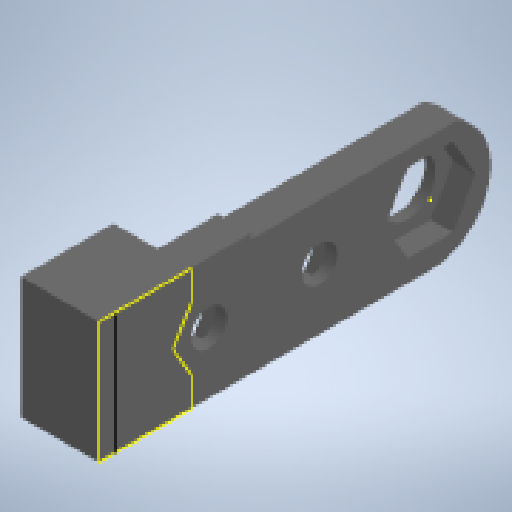
# Autodesk Inventor part: hand_finger_inside
Saved by Autodesk Inventor 2024.1 (Build 281209000, 209)
## iProperties
Created: 2025-01-23
Part Number: hand_finger_inside
Material: 一般
Document SubType Name: Modeling
Designer: hibik
Density: 1 g/cm^3
Appearance: 既定
Author: hibik
Autodesk Inventor part; units mm, degrees
ref_plane "YZ Plane" through (0, 0, 0) normal (1, 0, 0) x (0, 1, 0)
ref_plane "XZ Plane" through (0, 0, 0) normal (0, 1, 0) x (-1, 0, 0)
ref_plane "XY Plane" through (0, 0, 0) normal (0, 0, 1) x (1, 0, 0)
sketch "スケッチ1" plane through (0, 0, 0) normal (1, 0, 0) x (0, 1, 0)
  circle A0 centre (0, 0) radius 2.5
  line L0 (0, 4.0992) -> (3.55, 2.0496)
  line L1 (3.55, 2.0496) -> (3.55, -2.0496)
  line L2 (3.55, -2.0496) -> (0, -4.0992)
  line L3 (0, -4.0992) -> (-3.55, -2.0496)
  line L4 (-3.55, -2.0496) -> (-3.55, 2.0496)
  line L5 (-3.55, 2.0496) -> (0, 4.0992)
  circle A1 centre (0, 0) radius 5.5
  line L6 (5.5, 0) -> (-5.5, 0) construction
  line L7 (-5.5, 0) -> (-5.5, 30)
  line L8 (-5.5, 30) -> (5.5, 30)
  line L9 (5.5, 30) -> (5.5, 0)
  dimension "d2" = 11
  dimension "d0" = 5
  dimension "d1" = 7.1
  dimension "d3" = 30
  constraints: 20 end point, 3 coincident, 3 vertical, 2 parallel, 1 centre point, 1 horizontal, 1 perpendicular, 16 other
  measures "d0" diameter of A0
  measures "d1" distance between parallel lines of L4 L1
  measures "d3" distance of L8.end L6.start
extrude "押し出し1" add sketch "スケッチ1" along normal blind 3 contours A1 | A1 L7 L8 L9
extrude "押し出し2" add sketch "スケッチ1" along normal blind 1 contours L0 L1 L2 L3 L4 L5
sketch "スケッチ2" plane through (3, 0, 0) normal (1, 0, 0) x (0, 0, -1)
  circle A0 centre (-10, 0) radius 1.6
  circle A1 centre (-20, 0) radius 1.6
  point P0 (0, 0)
  dimension "d8" = 3.2
  dimension "d9" = 3.2
  dimension "d10" = 10
  dimension "d11" = 10
  constraints: 2 centre point, 2 horizontal alignment
  measures "d8" diameter of A0
  measures "d9" diameter of A1
  measures "d10" distance of point (0, 0) A0.centre
  measures "d11" distance of A1.centre A0.centre
extrude "押し出し3" cut sketch "スケッチ2" against normal through all
sketch "スケッチ3" plane through (0, 0, 0) normal (-1, 0, 0) x (0, 0, 1)
  circle A0 centre (20, 0) radius 1.6 projected
  circle A1 centre (10, 0) radius 1.6 projected
  line L0 (21.6454, -2.85) -> (18.3546, -2.85)
  line L1 (18.3546, -2.85) -> (16.7091, 0)
  line L2 (16.7091, 0) -> (18.3546, 2.85)
  line L3 (18.3546, 2.85) -> (21.6454, 2.85)
  line L4 (21.6454, 2.85) -> (23.2909, 0)
  line L5 (23.2909, 0) -> (21.6454, -2.85)
  line L6 (11.6454, -2.85) -> (8.3546, -2.85)
  line L7 (8.3546, -2.85) -> (6.7091, 0)
  line L8 (6.7091, 0) -> (8.3546, 2.85)
  line L9 (8.3546, 2.85) -> (11.6454, 2.85)
  line L10 (11.6454, 2.85) -> (13.2909, 0)
  line L11 (13.2909, 0) -> (11.6454, -2.85)
  point P0 (0, 0)
  dimension "d14" = 5.7
  constraints: 24 end point, 2 coincident, 2 horizontal, 1 point on line, 26 other
  measures "d14" distance between parallel lines of L3 L0
extrude "押し出し4" cut sketch "スケッチ3" against normal blind 2
sketch "スケッチ4" plane through (0, 0, 0) normal (-1, 0, 0) x (0, 0, 1)
  line L0 (16.2, 5) -> (-2.2913, 5) projected
  line L1 (16.2, 5.5) -> (16.2, 5) projected
  arc A0 (21.2458, 6.2407) -> (21.5454, 6.0705) centre (23.8648, 10.5) ccw projected
  line L2 (21.5454, 6.0705) -> (16.2, 6.0705)
  line L3 (16.2, 6.0705) -> (16.2, 5.8705)
  line L4 (16.2, 5.8705) -> (21.5454, 5.8705)
  line L5 (21.5454, 5.8705) -> (21.5454, 6.0705)
  arc A1 (0, 5.5) -> (0, -5.5) centre (0, 0) ccw projected
  line L6 (0, 5.5) -> (30, 5.5) projected
  point P0 (30, 5.5)
  point P1 (16.2, 5.3)
  dimension "d17" = 0.2
  constraints: 8 end point, 2 parallel, 1 collinear, 1 horizontal, 1 perpendicular, 1 other
  measures "d17" distance of L4.end L2.start
extrude "押し出し5" cut sketch "スケッチ4" against normal through all
sketch "スケッチ5" plane through (0, 0, 0) normal (-1, 0, 0) x (0, 0, 1)
  line L0 (23.2909, 0) -> (21.6454, -2.85) projected
  line L1 (21.6454, 2.85) -> (23.2909, 0) projected
  line L2 (30, -5.5) -> (0, -5.5) projected
  line L3 (21.6454, -5.5) -> (21.6454, 5.5)
  line L4 (16.2, 5.5) -> (30, 5.5) projected
  line L5 (23.8648, 5.5) -> (23.8648, 5.3) projected
  line L6 (30, 5.5) -> (30, -5.5) projected
  line L7 (30, 5.5) -> (16.1, 5.5) projected
  point P0 (0, 0)
  constraints: 3 point on line, 2 end point, 1 vertical
extrude "押し出し6" add sketch "スケッチ5" along normal blind 4 contours L1 L3 L4 L6 L2 L0
sketch "スケッチ7" plane through (-4, 0, 0) normal (-1, 0, 0) x (0, 0, 1)
  line L0 (30, 5.5) -> (21.6454, 5.5) projected
  line L1 (21.6454, 5.5) -> (21.6454, 2.85) projected
  line L2 (21.6454, 2.85) -> (23.2909, 0) projected
  line L3 (23.2909, 0) -> (21.6454, -2.85) projected
  line L4 (21.6454, -2.85) -> (21.6454, -5.5) projected
  line L5 (21.6454, -5.5) -> (30, -5.5) projected
  line L6 (30, -5.5) -> (30, 5.5) projected
  point P0 (0, 0)
extrude "押し出し7" add sketch "スケッチ7" against normal blind 10
sketch "スケッチ8" plane through (0, -5.5, 0) normal (0, -1, 0) x (1, 0, 0)
  circle A0 centre (3.5, 27) radius 1.6
  circle A1 centre (-1.5, 27) radius 1.6
  line L0 (6, 30) -> (6, 21.6454) projected
  line L1 (-4, 21.6454) -> (-4, 30) projected
  line L2 (-4, 30) -> (6, 30) projected
  point P0 (0, 0)
  dimension "d24" = 3.2
  dimension "d25" = 3.2
  dimension "d26" = 2.5
  dimension "d27" = 2.5
  dimension "d28" = 3
  constraints: 2 centre point, 1 horizontal alignment
  measures "d24" diameter of A0
  measures "d25" diameter of A1
  measures "d26" distance from line of L0 A0.centre
  measures "d27" distance from line of L1 A1.centre
  measures "d28" distance from line of L2 A0.centre
extrude "押し出し8" cut sketch "スケッチ8" against normal through all
equation "\"d11\" = d10"
equation "\"d27\" = d26"
